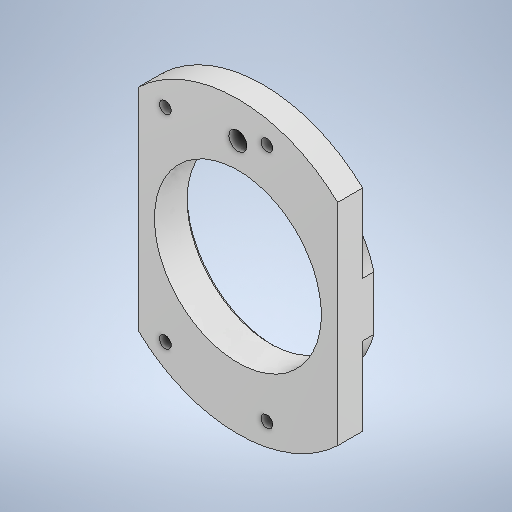
# Autodesk Inventor part: 27-30-400 Bearing, Housing Measuring Head
Saved by Autodesk Inventor 2025 (Build 290162000, 162)
## iProperties
Created: 2025-01-02
Part Number: 27-30-400 Bearing, Housing Measuring Head
Material: Aluminium
Document SubType Name: Modeling
Designer: marco.benkert
Density: 2.7 g/cm^3
Appearance: Satin
Author: marco.benkert
Autodesk Inventor part; units mm, degrees
ref_plane "YZ Plane" through (0, 0, 0) normal (1, 0, 0) x (0, 1, 0)
ref_plane "XZ Plane" through (0, 0, 0) normal (0, 1, 0) x (-1, 0, 0)
ref_plane "XY Plane" through (0, 0, 0) normal (0, 0, 1) x (1, 0, 0)
sketch "Skizze1" plane through (0, 0, 0) normal (0, 1, 0) x (-1, 0, 0)
  line L0 (-27.5, 29.0474) -> (-27.5, -29.0474)
  line L1 (27.5, -29.0474) -> (27.5, 29.0474)
  arc A0 (27.5, 29.0474) -> (-27.5, 29.0474) centre (0, 0) ccw
  arc A1 (-27.5, -29.0474) -> (27.5, -29.0474) centre (0, 0) ccw
  dimension "d4" = 27.5
  dimension "d5" = 40
  constraints: 4 end point, 4 point on circle, 2 centre point, 1 coincident, 1 parallel
  measures "d4" distance from line of point (0, 0) L1
  measures "d5" radius of A1
extrude "Basebody 1" add sketch "Skizze1" along normal blind 6.9
sketch "Skizze2" plane through (0, 6.9, 0) normal (0, 1, 0) x (1, 0, 0)
  line L0 (-27.5, 29.0474) -> (-27.5, -29.0474) projected
  arc A0 (27.5, 29.0474) -> (-27.5, 29.0474) centre (0, 0) ccw projected
  line L1 (-27.5, -7.4833) -> (-27.5, 7.4833)
  arc A1 (-27.5, -29.0474) -> (27.5, -29.0474) centre (0, 0) ccw projected
  line L2 (27.5, -7.4833) -> (27.5, 7.4833)
  arc A2 (-27.5, -7.4833) -> (27.5, -7.4833) centre (0, 0) ccw
  arc A3 (27.5, 7.4833) -> (-27.5, 7.4833) centre (0, 0) ccw
  constraints: 4 end point, 4 point on circle, 2 centre point, 2 vertical, 1 coincident
extrude "Basebody 2" add sketch "Skizze2" along normal blind 3.1
sketch "Skizze3" plane through (0, 10, 0) normal (0, 1, 0) x (1, 0, 0)
  arc A0 (27.5, 29.0474) -> (-27.5, 29.0474) centre (0, 0) ccw projected
  circle A1 centre (0, 0) radius 23
  dimension "d11" = 46
  constraints: 1 centre point, 1 coincident
  measures "d11" diameter of A1
extrude "42H7 Drill" cut sketch "Skizze3" against normal through all
sketch "Skizze4" plane through (0, 0, 0) normal (0, 1, 0) x (-1, 0, 0)
  circle A0 centre (0, 30) radius 2.5
  arc A1 (27.5, 7.4833) -> (-27.5, 7.4833) centre (0, 0) ccw projected
  dimension "d14" = 30
  dimension "d15" = 5
  constraints: 1 centre point
  measures "d14" distance of A1.centre A0.centre
  measures "d15" diameter of A0
extrude "5H7 Drill" cut sketch "Skizze4" along normal through all
sketch "Skizze6" plane through (0, 0, 0) normal (0, 1, 0) x (-1, 0, 0)
  circle A0 centre (20, 28) radius 2
  line L0 (-27.5, 29.0474) -> (-27.5, -29.0474) projected
  circle A1 centre (-8, 33) radius 2
  line L1 (32.1852, 0) -> (-31.2523, 0)
  circle A2 centre (20, -28) radius 2
  circle A3 centre (-8, -33) radius 2
  point P0 (0, 0)
  dimension "d18" = 4
  dimension "d19" = 28
  dimension "d20" = 47.5
  dimension "d21" = 4
  dimension "d22" = 33
  dimension "d23" = 19.5
  constraints: 4 centre point, 2 end point, 2 symmetric about line, 1 horizontal, 2 other
  measures "d18" diameter of A0
  measures "d19" vertical distance of point (0, 0) A0.centre
  measures "d20" distance from line of L0 A0.centre
  measures "d21" diameter of A1
  measures "d22" vertical distance of point (0, 0) A1.centre
  measures "d23" distance from line of L0 A1.centre
hole "M4" at (8, 0, 33) at (-20, 0, 28) at (-20, 0, -28) at (8, 0, -33) direction (0, 1, 0) diameter 3.242 end through all thread size "M4x0.7" class "6H" standard "ISO Metric profile"
chamfer "Fasen2" distance 1 angle 45 1 edges at (-23, 10, 0)
